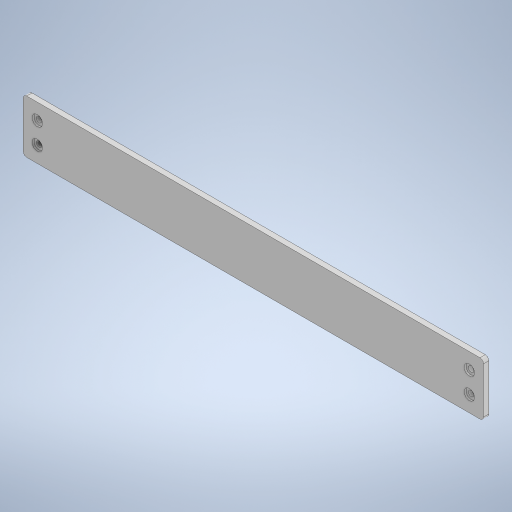
# Autodesk Inventor part: BP_BOX-Support-Bar
Saved by Autodesk Inventor 2024.3 (Build 283343000, 343)
## iProperties
Created: 2025-11-18
Part Number: BP_BOX-Support-Bar
Material: 一般
Document SubType Name: Modeling
Designer: 佐藤智貴
Density: 1 g/cm^3
Appearance: 既定
Author: 佐藤智貴
Autodesk Inventor part; units mm, degrees
ref_plane "YZ Plane" through (0, 0, 0) normal (1, 0, 0) x (0, 1, 0)
ref_plane "XZ Plane" through (0, 0, 0) normal (0, 1, 0) x (-1, 0, 0)
ref_plane "XY Plane" through (0, 0, 0) normal (0, 0, 1) x (1, 0, 0)
sketch "スケッチ1" plane through (0, 0, 0) normal (0, 0, 1) x (1, 0, 0)
  line L0 (0, 0) -> (260, 0)
  line L1 (260, 0) -> (260, 30)
  line L2 (260, 30) -> (0, 30)
  line L3 (0, 30) -> (0, 0)
  line L4 (0, 15) -> (260, 15)
  circle A0 centre (8, 21) radius 1.6
  circle A1 centre (8, 9) radius 1.6
  circle A2 centre (252, 21) radius 1.6
  circle A3 centre (252, 9) radius 1.6
  point P0 (8, 15)
  point P1 (252, 15)
  dimension "d0" = 260
  dimension "d1" = 244
  dimension "d2" = 8
  dimension "d3" = 30
  dimension "d4" = 15
  dimension "d5" = 9
  dimension "d6" = 9
  dimension "d7" = 9
  dimension "d8" = 9
  dimension "d9" = 3.2
  dimension "d10" = 3.2
  dimension "d11" = 3.2
  dimension "d12" = 3.2
  constraints: 10 end point, 4 centre point, 4 coincident, 2 midpoint, 2 parallel, 1 horizontal, 1 perpendicular
  measures "d0" distance of L1.end L2.end
  measures "d1" distance of point (252, 15) point (8, 15)
  measures "d2" distance from line of L3 point (8, 15)
  measures "d3" distance of L0.end L1.end
  measures "d4" distance from line of L0 point (8, 15)
  measures "d5" distance from line of L2 point (8, 21)
  measures "d6" distance from line of L0 point (8, 9)
  measures "d7" distance from line of L2 point (252, 21)
  measures "d8" distance from line of L0 point (252, 9)
  measures "d9" diameter of A0
  measures "d10" diameter of A1
  measures "d11" diameter of A2
  measures "d12" diameter of A3
extrude "押し出し1" add sketch "スケッチ1" along normal blind 3
sketch "スケッチ2" plane through (0, 0, 3) normal (0, 0, 1) x (1, 0, 0)
  line L0 (0, 30) -> (0, 0) projected
  line L1 (0, 0) -> (260, 0) projected
  line L2 (260, 0) -> (260, 30) projected
  line L3 (260, 30) -> (0, 30) projected
  circle A0 centre (8, 9) radius 1.6 projected
  circle A1 centre (252, 9) radius 1.6 projected
  circle A2 centre (252, 21) radius 1.6 projected
  circle A3 centre (8, 21) radius 1.6 projected
  circle A4 centre (8, 21) radius 3
  circle A5 centre (8, 9) radius 3
  circle A6 centre (252, 21) radius 3
  circle A7 centre (252, 9) radius 3
  dimension "d15" = 6
  dimension "d16" = 6
  dimension "d17" = 6
  dimension "d18" = 6
  constraints: 4 centre point
  measures "d15" diameter of A4
  measures "d16" diameter of A5
  measures "d17" diameter of A6
  measures "d18" diameter of A7
extrude "押し出し2" cut sketch "スケッチ2" against normal blind 1 contours A1 | A4 | A5 | A6 | A7
fillet "フィレット1" radius 2 4 edges at (260, 30, 1.5) (260, 0, 1.5) (0, 30, 1.5) (0, 0, 1.5)
equation "\"d2\" = -0.5 * d1 + 0.5 * d0"
equation "\"d4\" = 0.5 * d3"
equation "\"d6\" = d5"
equation "\"d7\" = d5"
equation "\"d8\" = d7"
equation "\"d10\" = d9"
equation "\"d11\" = d9"
equation "\"d12\" = d11"
equation "\"d16\" = d15"
equation "\"d17\" = d16"
equation "\"d18\" = d17"
